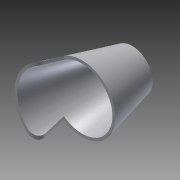
# Autodesk Inventor part: ball受け
Saved by Autodesk Inventor 2015 (Build 190159000, 159)
## iProperties
Created: 2015-05-15
Part Number: ball受け
Material: ABS プラスチック
Document SubType Name: Modeling
Designer: Shun
Density: 1.06 g/cm^3
Appearance: 滑らか - 白
Mass: 36.5553 g
Surface Area: 237.934 cm^2
Volume: 34.4861 cm^3
Author: Shun
Autodesk Inventor part; units mm, degrees
ref_plane "YZ Plane" through (0, 0, 0) normal (1, 0, 0) x (0, 1, 0)
ref_plane "XZ Plane" through (0, 0, 0) normal (0, 1, 0) x (-1, 0, 0)
ref_plane "XY Plane" through (0, 0, 0) normal (0, 0, 1) x (1, 0, 0)
sketch "スケッチ8" plane through (0, 0, 0) normal (0, 0, 1) x (1, 0, 0)
  line L0 (0, 0) -> (0, 85)
  line L1 (0, 85) -> (22.5, 85)
  line L2 (22.5, 85) -> (44, 0)
  line L3 (44, 0) -> (0, 0)
  dimension "d14" = 22.5
  dimension "d15" = 44
  dimension "d16" = 85
  constraints: 8 end point, 1 parallel, 1 perpendicular, 1 vertical
  measures "d14" distance of L0.end L1.end
  measures "d15" distance of L2.end L0.start
  measures "d16" distance of L0.start L0.end
revolve "回転1" add sketch "スケッチ8" angle 360 about axis through (0, 0, 0) along (0, 1, 0)
shell "シェル2" thickness 3 removed faces 1 at (-13.3987, 0, -0.1333)
sketch "スケッチ9" plane through (0, 82, 0) normal (0, -1, 0) x (1, 0, 0)
  circle A0 centre (0, 0) radius 1.5
  dimension "d29" = 3
  constraints: 1 centre point, 1 coincident
  measures "d29" diameter of A0
hole "穴2" at (0, 82, 0) direction (0, 1, 0) diameter 3 end through all
sketch "スケッチ16" plane through (0, 0, 0) normal (0, -1, 0) x (1, 0, 0)
  line L0 (80, -50) -> (-20, -50)
  line L1 (-20, -50) -> (-20, 50)
  line L2 (-20, 50) -> (80, 50)
  line L3 (80, 50) -> (80, -50)
  point P0 (0, 0)
  dimension "d66" = 100
  dimension "d67" = 100
  dimension "d68" = 50
  dimension "d69" = 20
  constraints: 8 end point, 2 parallel, 1 horizontal, 1 perpendicular
  measures "d66" distance of L1.end L2.end
  measures "d67" distance of L0.end L1.end
  measures "d68" distance from line of L0 point (0, 0)
  measures "d69" distance from line of L1 point (0, 0)
extrude "押し出し6" cut sketch "スケッチ16" against normal blind 30
fillet "フィレット3" radius 10 2 edges at (-20, 0, -37.4373) (-20, 0, 37.4373)
sketch "スケッチ17" plane through (0, 82, 0) normal (0, -1, 0) x (1, 0, 0)
  line L0 (0, 0) -> (-4.2426, -4.2426)
  line L1 (0, 0) -> (6, 0) construction
  circle A0 centre (-4.2426, -4.2426) radius 1.25
  dimension "d73" = 6
  dimension "d74" = 135
  dimension "d75" = 2.5
  constraints: 4 end point, 1 centre point, 1 coincident, 1 equal length, 1 horizontal
  measures "d73" distance of L0.start L0.end
  measures "d74" angle of L0 L1
  measures "d75" diameter of A0
extrude "押し出し7" cut sketch "スケッチ17" against normal blind 30
pattern_circular "円形状パターン2" count 4 over 360 about axis through (0, 232.7083, 0) along (0, -1, 0) of "押し出し7"
